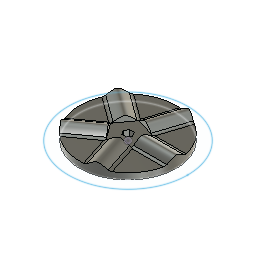
disc_up_down (Autodesk Fusion 360 design; units mm, degrees)
part number: 2026-05-12-14-40-25-549
Autodesk Fusion 360 part; units mm, degrees
note: some values were not read from the file. Chosen so that the rebuilt part matches the saved one: which pieces of a blend or face edit are solid.
sketch "Sketch3" plane through (0, 0, 0) normal (0, 0, 1) x (1, 0, 0)
  circle A0 centre (0, 0) radius 49.5
  circle A1 centre (0, 0) radius 61.1953
  dimension "d4" = 99
  constraint coincident A0.centre A1.centre
  constraint concentric A0 A1
  measures "d4" diameter of A0
extrude "Extrude2" add sketch "Sketch3" along normal blind 6.5 contours A0
ref_plane "WorkPlane1" through (49.5, 0, 2.7519) normal (1, 0, 0) x (0, -1, 0)
sketch "Sketch4" plane through (49.5, 0, 0) normal (1, 0, 0) x (0, 1, 0)
  line L0 (49.5, 6.5) -> (-49.5, 6.5)
  spline S0 degree 2 poles (9.9609, 6.5) (0, 14) (-10.0579, 6.5) knots 0 0 0 2.29633 2.29633 2.29633 weights 1 3 1
  constraint coincident L0 S0.end
  constraint coincident L0 S0.start
extrude "Extrude3" add sketch "Sketch4" against normal blind 35
pattern_circular "C-Pattern1" count 5 over 360 about axis through (0, 0, -11.25) along (0, 0, 1) of "Extrude3"
extrude "Extrude4" cut sketch "Sketch3" along normal blind 30
fillet "Fillet1" radius 5 1 edges at (-19.6241, -26.57, 6.5)
fillet "Fillet1" radius 5 9 edges at (-31.3827, -10.3687, 6.5) (-31.3338, 10.453, 6.5) (-19.559, 26.6426, 6.5) (0.2588, 33.0304, 6.5) (19.2946, 26.8347, 6.5) (31.4937, 9.9609, 6.5) (31.4837, -10.0579, 6.5) (19.2054, -26.8742, 6.5) (0.1634, -33.0508, 6.5)
sketch "Sketch6" plane through (0, 0, 6.5) normal (0, 0, 1) x (-1, 0, 0)
  line L0 (5.5385, 17.0458) -> (-14.5, 10.5349)
  line L1 (-14.5, 10.5349) -> (-14.5, -10.5349)
  line L2 (-14.5, -10.5349) -> (5.5385, -17.0458)
  line L3 (5.5385, -17.0458) -> (17.923, 0)
  line L4 (17.923, 0) -> (5.5385, 17.0458)
  line L5 (-2.4696, 4.116) -> (-4.7993, -0.0807)
  line L6 (-4.7993, -0.0807) -> (-2.3297, -4.1967)
  line L7 (-2.3297, -4.1967) -> (2.4696, -4.116)
  line L8 (2.4696, -4.116) -> (4.7993, 0.0807)
  line L9 (4.7993, 0.0807) -> (2.3297, 4.1967)
  line L10 (2.3297, 4.1967) -> (-2.4696, 4.116)
  dimension "d19" = 4.8
  measures "d19" distance of L5.start origin
extrude "Extrude5" cut sketch "Sketch6" against normal blind 15 contours L5 L6 L7 L8 L9 L10
sketch "Sketch1" plane through (0, 0, 0) normal (1, 0, 0) x (0, 1, 0)
  circle A0 centre (0, 30) radius 25
  dimension "d1" = 50
  measures "d1" diameter of A0
extrude "Extrude1" [suppressed]
sketch "Sketch2" plane through (0, 0, 0) normal (1, 0, 0) x (0, 1, 0)
  line L0 (130, 170) -> (140.9808, 210.9808)
  line L1 (140.9808, 210.9808) -> (110.9808, 240.9808)
  line L2 (110.9808, 240.9808) -> (70, 230)
  line L3 (70, 230) -> (59.0192, 189.0192)
  line L4 (59.0192, 189.0192) -> (89.0192, 159.0192)
  line L5 (89.0192, 159.0192) -> (130, 170)
  point P0 (100, 200)
